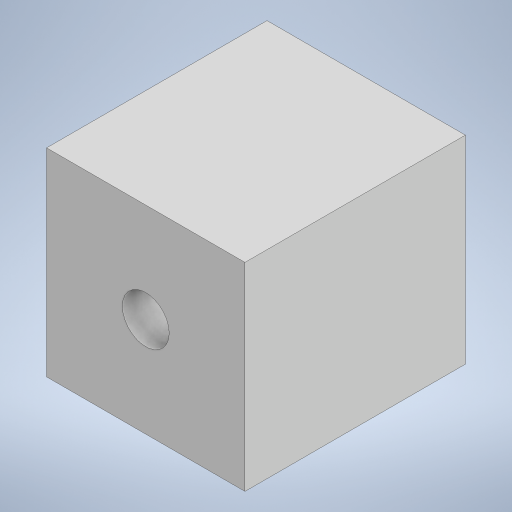
# Autodesk Inventor part: Motor
Saved by Autodesk Inventor 2024 (Build 280153000, 153)
## iProperties
Created: 2024-05-15
Part Number: Motor
Material: Generisch
Document SubType Name: Modeling
Designer: month
Density: 1 g/cm^3
Appearance: Vorgabe
Author: month
Autodesk Inventor part; units mm, degrees
ref_plane "YZ Plane" through (0, 0, 0) normal (1, 0, 0) x (0, 1, 0)
ref_plane "XZ Plane" through (0, 0, 0) normal (0, 1, 0) x (-1, 0, 0)
ref_plane "XY Plane" through (0, 0, 0) normal (0, 0, 1) x (1, 0, 0)
sketch "Skizze1" plane through (0, 0, 0) normal (0, 1, 0) x (-1, 0, 0)
  line L0 (0, 0) -> (42.3, 0)
  line L1 (42.3, 0) -> (42.3, -42.3)
  line L2 (42.3, -42.3) -> (0, -42.3)
  line L3 (0, -42.3) -> (0, 0)
  dimension "d0" = 42.3
  dimension "d1" = 42.3
  constraints: 8 end point, 2 parallel, 1 horizontal, 1 perpendicular
  measures "d0" distance of L2.end L0.start
  measures "d1" distance of L1.end L2.end
extrude "Extrusion1" add sketch "Skizze1" along normal blind 47
sketch "Skizze2" plane through (0, 47, 0) normal (0, 1, 0) x (1, 0, 0)
  line L0 (-42.3, 42.3) -> (-42.3, 0) projected
  line L1 (-42.3, 21.15) -> (0, 21.15)
  line L2 (0, 0) -> (0, 42.3) projected
  line L3 (-42.3, 0) -> (0, 0) projected
  line L4 (-21.15, 0) -> (-21.15, 42.3)
  line L5 (0, 42.3) -> (-42.3, 42.3) projected
  circle A0 centre (-21.15, 21.15) radius 5
  dimension "d4" = 10
  constraints: 5 midpoint, 4 end point, 1 centre point
  measures "d4" diameter of A0
extrude "Extrusion2" cut sketch "Skizze2" against normal blind 47 contours A0 L4 L1 | L1 L4 A0 | A0 L1 L4 | L1 A0 L4
